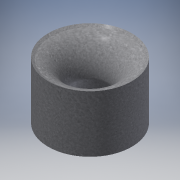
# Autodesk Inventor part: Graphite
Saved by Autodesk Inventor 2017 (Build 210142000, 142)
## iProperties
Created: 2016-01-09
Part Number: Graphite
Material: GFRC
Document SubType Name: Modeling
Designer: Jared
Density: 1.7 g/cm^3
Appearance: Flat - Polished Gray
Author: Jared
Autodesk Inventor part; units mm, degrees
ref_plane "YZ Plane" through (0, 0, 0) normal (1, 0, 0) x (0, 1, 0)
ref_plane "XZ Plane" through (0, 0, 0) normal (0, 1, 0) x (-1, 0, 0)
ref_plane "XY Plane" through (0, 0, 0) normal (0, 0, 1) x (1, 0, 0)
sketch "Sketch1" plane through (0, 0, 0) normal (0, 0, 1) x (1, 0, 0)
  arc A0 (-25.8327, -3.287) -> (-25.4, 0) centre (-38.1, 0) ccw
  line L0 (-59.2667, 42.6459) -> (-60.6149, 42.6459)
  line L1 (-59.2667, 42.6459) -> (0, 42.6459) construction
  line L2 (-41.4694, -37.9453) -> (-35.1194, -37.9453)
  line L3 (-80.7, -43.0791) -> (-21.9625, -43.0791) construction
  line L4 (-87.05, -219.9038) -> (-83.875, -219.9038)
  line L5 (0, 42.6459) -> (0, 0)
  line L6 (-87.8501, 55.3459) -> (-18.3062, 55.3459) construction
  line L7 (-87.8501, 55.3459) -> (-14.7047, 55.3459) construction
  line L8 (-87.8501, 55.3459) -> (-52.22, 55.3459) construction
  arc A1 (-25.4, 0) -> (-55.5582, 40.2879) centre (-67.3891, 0) ccw
  line L9 (-59.2667, 42.6459) -> (-59.2667, -37.9453)
  line L10 (-59.2667, 42.6459) -> (21.3245, 42.6459) construction
  line L11 (-59.2667, -37.9453) -> (-41.4694, -37.9453)
  line L12 (-55.5582, 40.2879) -> (-59.2667, 42.6459)
  line L13 (-35.1194, -37.9453) -> (-25.8327, -3.287)
  dimension "d56" = 25.4
  dimension "d60" = 12.7
  dimension "d61" = 12.7
  dimension "d62" = 59.2667
  dimension "d63" = 6.35
  dimension "d77" = 3.175
  dimension "d84" = 41.9891
  dimension "d85" = 32.2919
  dimension "d86" = 90
  dimension "d87" = 80.5912
  constraints: 29 end point, 9 horizontal, 4 point on circle, 3 horizontal alignment, 3 perpendicular, 2 centre point, 1 other
  measures "d56" distance of A1.start L5.end
  measures "d60" vertical distance of L0.start L6.start
  measures "d61" radius of A0
  measures "d62" horizontal distance of L5.end L0.start
  measures "d63" distance of L2.start L2.end
  measures "d77" distance of L4.end L4.start
  measures "d84" radius of A1
  measures "d85" horizontal distance of L6.start L12.start
  measures "d86" angle of L9 L10
  measures "d87" distance of L0.start L11.start
revolve "Revolution1" add sketch "Sketch1" angle 360 about axis through (0, 42.6459, 0) along (0, -1, 0)
body "Solid1"
